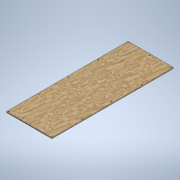
# Autodesk Inventor part: Cobertura
Saved by Autodesk Inventor 2020.2 (Build 242310000, 310)
## iProperties
Created: 2020-07-15
Part Number: Cobertura
Material: Wood (Oak)
Document SubType Name: Modeling
Designer: JK
Density: 0.76 g/cm^3
Appearance: Plywood - Weathered
Author: JK
Autodesk Inventor part; units mm, degrees
ref_plane "YZ Plane" through (0, 0, 0) normal (1, 0, 0) x (0, 1, 0)
ref_plane "XZ Plane" through (0, 0, 0) normal (0, 1, 0) x (-1, 0, 0)
ref_plane "XY Plane" through (0, 0, 0) normal (0, 0, 1) x (1, 0, 0)
sketch "Sketch1" plane through (0, 0, 0) normal (0, 1, 0) x (-1, 0, 0)
  line L0 (-280, 750) -> (280, 750)
  line L1 (280, 750) -> (280, -750)
  line L2 (280, -750) -> (-280, -750)
  line L3 (-280, -750) -> (-280, 750)
  line L4 (-280, 750) -> (280, -750) construction
  line L5 (280, 750) -> (-280, -750) construction
  point P0 (0, 0)
  dimension "d0" = 1500
  dimension "d1" = 560
  constraints: 12 end point, 2 midpoint, 2 parallel, 1 horizontal, 1 perpendicular
  measures "d0" distance of L0.end L1.end
  measures "d1" distance of L1.end L2.end
extrude "Extrusion1" add sketch "Sketch1" along normal blind 12.5
sketch "Sketch2" plane through (0, 12.5, 0) normal (0, 1, 0) x (1, 0, 0)
  circle A0 centre (-265, -735) radius 3
  line L0 (-280, 750) -> (-280, -750) projected
  line L1 (280, -750) -> (280, 750) projected
  line L2 (-280, -750) -> (280, -750) projected
  dimension "d4" = 6
  dimension "d5" = 15
  dimension "d7" = 15
  constraints: 1 centre point
  measures "d4" diameter of A0
  measures "d5" distance from line of L0 A0.centre
  measures "d7" distance from line of L2 A0.centre
extrude "Extrusion2" cut sketch "Sketch2" against normal through all
pattern_linear "Rectangular Pattern1" count 5 spacing 367.5 along (0, 0, -1) count 2 spacing 530 along (1, 0, 0) of "Extrusion2"
sketch "Sketch3" plane through (0, 12.5, 0) normal (0, 1, 0) x (1, 0, 0)
  circle A0 centre (0, -735) radius 3
  circle A1 centre (0, 735) radius 3
  line L0 (280, 750) -> (-280, 750) projected
  line L1 (-280, -750) -> (280, -750) projected
  point P0 (0, 0)
  dimension "d16" = 6
  dimension "d17" = 15
  dimension "d18" = 15
  dimension "d19" = 6
  constraints: 2 centre point
  measures "d16" diameter of A1
  measures "d17" distance from line of L0 A1.centre
  measures "d18" distance from line of L1 A0.centre
  measures "d19" diameter of A0
extrude "Extrusion3" cut sketch "Sketch3" against normal through all
sketch "Sketch4" plane through (0, 12.5, 0) normal (0, 1, 0) x (1, 0, 0)
  circle A0 centre (-265, -735) radius 3 projected
  circle A1 centre (-265, -735) radius 4.75
  point P0 (0, 0)
  dimension "d22" = 9.5
  constraints: 1 centre point, 1 coincident
  measures "d22" diameter of A1
extrude "Extrusion4" cut sketch "Sketch4" against normal blind 2 contours A0 | A1
pattern_linear "Rectangular Pattern2" count 5 spacing 367.5 along (0, 0, -1) count 2 spacing 530 along (1, 0, 0) of "Extrusion4"
sketch "Sketch5" plane through (0, 12.5, 0) normal (0, 1, 0) x (1, 0, 0)
  circle A0 centre (0, -735) radius 3 projected
  circle A1 centre (0, -735) radius 4.75
  circle A2 centre (0, 735) radius 3 projected
  circle A3 centre (0, 735) radius 4.75
  point P0 (0, 0)
  dimension "d31" = 9.5
  dimension "d32" = 9.5
  constraints: 2 centre point, 2 coincident
  measures "d31" diameter of A3
  measures "d32" diameter of A1
extrude "Extrusion5" cut sketch "Sketch5" against normal blind 2 contours A0 | A1 | A2 | A3
body "Solid1"
